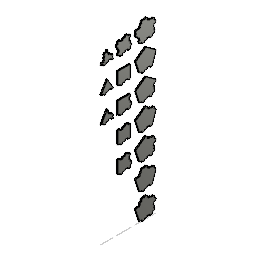
Test Game Pieces v1 (Autodesk Fusion 360 design; units mm, degrees)
Autodesk Fusion 360 part; units mm, degrees
sketch "Sketch1" plane through (0, 0, 0) normal (1, 0, 0) x (0, 0, -1)
  line L0 (0, 0) -> (10, 0)
  line L1 (5, 0) -> (5, 1)
  line L2 (5, 1) -> (5, 15)
  line L3 (10, 0) -> (5, 8.6603)
  line L4 (5, 8.6603) -> (0, 0)
  dimension "d1" = 10
  dimension "d2" = 10
  constraint coincident L0.start L4.end
  constraint horizontal L0
  constraint midpoint L0 L1.start
  constraint perpendicular L0 L1
  constraint perpendicular L0 L2
  constraint coincident L2 L3.end
  measures "d1" distance of L0.start L0.end
  measures "d2" distance of L0.end L3.end
extrude "Extrude1" add sketch "Sketch1" along normal blind 1 makes body 1
sketch "Sketch2" plane through (0, 0, 0) normal (1, 0, 0) x (0, 0, -1)
  line L0 (15, 0) -> (25, 0)
  line L1 (25, 0) -> (25, 10)
  line L2 (25, 10) -> (15, 10)
  line L3 (15, 10) -> (15, 0)
  dimension "d5" = 10
  dimension "d6" = 10
  constraint horizontal L0
  constraint vertical L1
  constraint horizontal L2
  constraint vertical L3
  measures "d5" distance of L0.start L0.end
  measures "d6" distance of L0.start L2.end
extrude "Extrude2" add sketch "Sketch2" along normal blind 1 separate body makes body 2
sketch "Sketch3" plane through (0, 0, 0) normal (1, 0, 0) x (0, 0, -1)
  line L0 (30, 0) -> (40, 0)
  line L1 (40, 0) -> (43.0902, 9.5106)
  line L2 (40, 0) -> (50, 0) construction
  line L3 (43.0902, 9.5106) -> (35, 15.3884)
  line L4 (43.0902, 9.5106) -> (53.0902, 9.5106) construction
  line L5 (30, 0) -> (26.9098, 9.5106)
  line L6 (30, 0) -> (40, 0) construction
  line L7 (26.9098, 9.5106) -> (35, 15.3884)
  dimension "d9" = 10
  dimension "d10" = 72
  dimension "d11" = 10
  dimension "d12" = 144
  dimension "d13" = 10
  dimension "d14" = 108
  dimension "d15" = 10
  constraint horizontal L0
  constraint horizontal L2
  constraint horizontal L4
  constraint horizontal L6
  measures "d9" distance of L0.start L0.end
  measures "d10" angle of L1 L2
  measures "d11" distance of L0.end L1.end
  measures "d12" angle of L3 L4
  measures "d13" distance of L1.end L3.end
  measures "d14" angle of L5 L6
  measures "d15" distance of L0.start L5.end
extrude "Extrude3" add sketch "Sketch3" along normal blind 1 separate body makes body 3
move_body "Move1" bodies 2 to x (1, 0, 0) y (0, 1, 0) z (0, 0, 1) at (0, 0, 2)
sketch "Sketch4" plane through (1, 0, 0) normal (1, 0, 0) x (0, 0, -1)
  line L0 (5, 8.6603) -> (0, 0)
  line L1 (0, 0) -> (10, 0)
  line L2 (10, 0) -> (5, 8.6603)
  line L3 (5, 0) -> (6, 0)
  line L4 (5, 0) -> (4, 0)
  line L5 (4, 0) -> (2, 0)
  line L6 (2, 0) -> (2, -1)
  line L7 (2, -1) -> (4, -1)
  line L8 (4, -1) -> (4, 0)
  line L9 (6, 0) -> (8, 0)
  line L10 (8, 0) -> (8, 1)
  line L11 (8, 1) -> (6, 1)
  line L12 (6, 1) -> (6, 0)
  line L13 (7.5, 4.3301) -> (8, 3.4641)
  line L14 (7.5, 4.3301) -> (7, 5.1962)
  line L15 (7, 5.1962) -> (6.134, 4.6962)
  line L16 (7, 5.1962) -> (6, 6.9282)
  line L17 (6, 6.9282) -> (5.134, 6.4282)
  line L18 (5.134, 6.4282) -> (6.134, 4.6962)
  line L19 (8, 3.4641) -> (8.866, 3.9641)
  line L20 (8.866, 3.9641) -> (9.866, 2.2321)
  line L21 (9.866, 2.2321) -> (9, 1.7321)
  line L22 (2.5, 4.3301) -> (3, 5.1962)
  line L23 (3, 5.1962) -> (2.134, 5.6962)
  line L24 (2.134, 5.6962) -> (3.134, 7.4282)
  line L25 (3.134, 7.4282) -> (4, 6.9282)
  line L26 (2.5, 4.3301) -> (2, 3.4641)
  line L27 (2, 3.4641) -> (2.866, 2.9641)
  line L28 (2.866, 2.9641) -> (1.866, 1.2321)
  line L29 (1.866, 1.2321) -> (1, 1.7321)
  dimension "d18" = 1
  dimension "d19" = 1
  dimension "d20" = 1
  dimension "d21" = 2
  dimension "d22" = 1
  dimension "d23" = 1
  dimension "d24" = 1
  dimension "d25" = 1
  dimension "d26" = 2
  dimension "d27" = 1
  dimension "d28" = 1
  dimension "d29" = 2
  dimension "d30" = 1
  dimension "d31" = 1
  dimension "d32" = 2
  dimension "d33" = 1
  dimension "d34" = 1
  dimension "d35" = 2
  constraint midpoint L1 L3.start
  constraint parallel L1 L3
  constraint parallel L1 L4
  constraint horizontal L5
  constraint vertical L6
  constraint horizontal L7
  constraint vertical L8
  constraint horizontal L9
  constraint vertical L10
  constraint horizontal L11
  constraint vertical L12
  constraint midpoint L2 L13.start
  constraint parallel L2 L13
  constraint parallel L2 L14
  constraint perpendicular L2 L15
  constraint perpendicular L15 L16
  constraint perpendicular L2 L17
  constraint perpendicular L13 L19
  constraint perpendicular L19 L20
  constraint coincident L2 L21.end
  constraint perpendicular L2 L21
  constraint midpoint L0 L22.start
  constraint parallel L0 L22
  constraint perpendicular L0 L23
  constraint perpendicular L23 L24
  constraint coincident L0 L25.end
  constraint perpendicular L0 L25
  constraint perpendicular L23 L26
  constraint perpendicular L0 L27
  constraint perpendicular L27 L28
  constraint coincident L0 L29.end
  constraint perpendicular L0 L29
  measures "d18" distance of L3.start L3.end
  measures "d19" distance of L3.start L4.end
  measures "d20" distance of L4.end L7.end
  measures "d21" distance of L3.end L9.end
  measures "d22" distance of L3.end L11.end
  measures "d23" distance of L13.start L13.end
  measures "d24" distance of L13.start L14.end
  measures "d25" distance of L14.end L15.end
  measures "d26" distance of L14.end L16.end
  measures "d27" distance of L16.end L17.end
  measures "d28" distance of L13.end L19.end
  measures "d29" distance of L19.end L20.end
  measures "d30" distance of L22.start L22.end
  measures "d31" distance of L22.end L23.end
  measures "d32" distance of L23.end L24.end
  measures "d33" distance of L22.start L26.end
  measures "d34" distance of L26.end L27.end
  measures "d35" distance of L27.end L28.end
extrude "Extrude4" add sketch "Sketch4" against normal blind 1 contours L1 L5 L6 L7 L8 bodies 1
extrude "Extrude5" cut sketch "Sketch4" against normal blind 1 contours L1 L9 L10 L11 L12 bodies 1
copy_body "CopyPasteBodies1" bodies 1 makes body 4
move_body "Move2" bodies 4 to x (1, 0, 0) y (0, 1, 0) z (0, 0, 1) at (0, -20, 0)
extrude "Extrude6" cut sketch "Sketch4" against normal blind 1 contours L2 L15 L16 L17 L18 bodies 1
extrude "Extrude7" add sketch "Sketch4" against normal blind 1 contours L2 L19 L20 L21 bodies 1
copy_body "CopyPasteBodies2" bodies 1 makes body 5
move_body "Move3" bodies 5 to x (1, 0, 0) y (0, 1, 0) z (0, 0, 1) at (0, -40, 0)
extrude "Extrude8" cut sketch "Sketch4" against normal blind 1 contours L0 L27 L28 L29 bodies 1
extrude "Extrude9" add sketch "Sketch4" against normal blind 1 contours L0 L23 L24 L25 bodies 1
sketch "Sketch5" plane through (1, 0, 0) normal (1, 0, 0) x (0, 0, -1)
  line L0 (13, 10) -> (13, 0)
  line L1 (13, 0) -> (23, 0)
  line L2 (23, 0) -> (23, 10)
  line L3 (23, 10) -> (13, 10)
  line L4 (18, 0) -> (19, 0)
  line L5 (19, 0) -> (21, 0)
  line L6 (21, 0) -> (21, 1)
  line L7 (21, 1) -> (19, 1)
  line L8 (19, 1) -> (19, 0)
  line L9 (18, 0) -> (17, 0)
  line L10 (17, 0) -> (15, 0)
  line L11 (15, 0) -> (15, -1)
  line L12 (15, -1) -> (17, -1)
  line L13 (17, -1) -> (17, 0)
  line L14 (23, 5) -> (23, 4)
  line L15 (23, 4) -> (24, 4)
  line L16 (24, 4) -> (24, 2)
  line L17 (24, 2) -> (23, 2)
  line L18 (23, 2) -> (23, 4)
  line L19 (23, 5) -> (23, 6)
  line L20 (23, 6) -> (22, 6)
  line L21 (22, 6) -> (22, 8)
  line L22 (22, 8) -> (23, 8)
  line L23 (23, 8) -> (23, 6)
  line L24 (18, 10) -> (19, 10)
  line L25 (19, 10) -> (21, 10)
  line L26 (21, 10) -> (21, 11)
  line L27 (21, 11) -> (19, 11)
  line L28 (19, 11) -> (19, 10)
  line L29 (18, 10) -> (17, 10)
  line L30 (17, 10) -> (15, 10)
  line L31 (15, 10) -> (15, 9)
  line L32 (15, 9) -> (17, 9)
  line L33 (17, 9) -> (17, 10)
  line L34 (13, 5) -> (13, 6)
  line L35 (13, 6) -> (12, 6)
  line L36 (12, 6) -> (12, 8)
  line L37 (12, 8) -> (13, 8)
  line L38 (13, 8) -> (13, 6)
  line L39 (13, 5) -> (13, 4)
  line L40 (13, 4) -> (14, 4)
  line L41 (14, 4) -> (14, 2)
  line L42 (14, 2) -> (13, 2)
  line L43 (13, 2) -> (13, 4)
  dimension "d48" = 1
  dimension "d49" = 2
  dimension "d50" = 1
  dimension "d51" = 1
  dimension "d52" = 2
  dimension "d53" = 1
  dimension "d54" = 1
  dimension "d55" = 1
  dimension "d56" = 2
  dimension "d57" = 1
  dimension "d58" = 1
  dimension "d59" = 2
  dimension "d60" = 1
  dimension "d61" = 2
  dimension "d62" = 1
  dimension "d63" = 1
  dimension "d64" = 2
  dimension "d65" = 1
  dimension "d66" = 1
  dimension "d67" = 1
  dimension "d68" = 2
  dimension "d69" = 1
  dimension "d70" = 1
  dimension "d71" = 2
  constraint midpoint L1 L4.start
  constraint parallel L1 L4
  constraint horizontal L5
  constraint vertical L6
  constraint horizontal L7
  constraint vertical L8
  constraint parallel L1 L9
  constraint horizontal L10
  constraint vertical L11
  constraint horizontal L12
  constraint vertical L13
  constraint midpoint L2 L14.start
  constraint parallel L2 L14
  constraint horizontal L15
  constraint vertical L16
  constraint horizontal L17
  constraint vertical L18
  constraint parallel L2 L19
  constraint horizontal L20
  constraint vertical L21
  constraint horizontal L22
  constraint vertical L23
  constraint midpoint L3 L24.start
  constraint parallel L3 L24
  constraint horizontal L25
  constraint vertical L26
  constraint horizontal L27
  constraint vertical L28
  constraint parallel L3 L29
  constraint horizontal L30
  constraint vertical L31
  constraint horizontal L32
  constraint vertical L33
  constraint midpoint L0 L34.start
  constraint parallel L0 L34
  constraint horizontal L35
  constraint vertical L36
  constraint horizontal L37
  constraint vertical L38
  constraint parallel L0 L39
  constraint horizontal L40
  constraint vertical L41
  constraint horizontal L42
  constraint vertical L43
  measures "d48" distance of L4.start L4.end
  measures "d49" distance of L4.end L5.end
  measures "d50" distance of L4.end L7.end
  measures "d51" distance of L4.start L9.end
  measures "d52" distance of L9.end L10.end
  measures "d53" distance of L9.end L12.end
  measures "d54" distance of L14.start L14.end
  measures "d55" distance of L14.end L15.end
  measures "d56" distance of L14.end L17.end
  measures "d57" distance of L14.start L19.end
  measures "d58" distance of L19.end L20.end
  measures "d59" distance of L19.end L22.end
  measures "d60" distance of L24.start L24.end
  measures "d61" distance of L24.end L25.end
  measures "d62" distance of L24.end L27.end
  measures "d63" distance of L24.start L29.end
  measures "d64" distance of L29.end L30.end
  measures "d65" distance of L29.end L32.end
  measures "d66" distance of L34.start L34.end
  measures "d67" distance of L34.end L35.end
  measures "d68" distance of L34.end L37.end
  measures "d69" distance of L34.start L39.end
  measures "d70" distance of L39.end L40.end
  measures "d71" distance of L39.end L42.end
extrude "Extrude10" add sketch "Sketch5" against normal blind 1 contours L1 L10 L11 L12 L13 bodies 2
extrude "Extrude11" cut sketch "Sketch5" against normal blind 1 contours L1 L5 L6 L7 L8 bodies 2
copy_body "CopyPasteBodies3" bodies 2 makes body 6
move_body "Move4" bodies 6 to x (1, 0, 0) y (0, 1, 0) z (0, 0, 1) at (0, -20, 0)
extrude "Extrude12" cut sketch "Sketch5" against normal blind 1 contours L2 L20 L21 L22 L23 bodies 2
extrude "Extrude13" add sketch "Sketch5" against normal blind 1 contours L2 L15 L16 L17 L18 bodies 2
copy_body "CopyPasteBodies4" bodies 2 makes body 7
move_body "Move5" bodies 7 to x (1, 0, 0) y (0, 1, 0) z (0, 0, 1) at (0, -40, 0)
extrude "Extrude14" cut sketch "Sketch5" against normal blind 1 contours L2 L15 L16 L17 L18 bodies 2
extrude "Extrude15" add sketch "Sketch5" against normal blind 1 contours L2 L20 L21 L22 L23 bodies 2
extrude "Extrude16" add sketch "Sketch5" against normal blind 1 contours L3 L25 L26 L27 L28 bodies 2
extrude "Extrude17" cut sketch "Sketch5" against normal blind 1 contours L3 L30 L31 L32 L33 bodies 2
copy_body "CopyPasteBodies5" bodies 2 makes body 8
move_body "Move6" bodies 8 to x (1, 0, 0) y (0, 1, 0) z (0, 0, 1) at (0, -60, 0)
extrude "Extrude18" add sketch "Sketch5" against normal blind 1 contours L3 L30 L31 L32 L33 bodies 2
extrude "Extrude19" cut sketch "Sketch5" against normal blind 1 contours L3 L25 L26 L27 L28 bodies 2
extrude "Extrude20" add sketch "Sketch5" against normal blind 1 contours L0 L35 L36 L37 L38 bodies 2
extrude "Extrude21" cut sketch "Sketch5" against normal blind 1 contours L0 L40 L41 L42 L43 bodies 2
extrude "Extrude22" cut sketch "Sketch5" against normal blind 1 contours L0 L35 L36 L37 L38 | L2 L20 L21 L22 L23 bodies 2
extrude "Extrude23" add sketch "Sketch5" against normal blind 1 contours L0 L40 L41 L42 L43 | L2 L15 L16 L17 L18 bodies 2
extrude "Extrude24" cut sketch "Sketch5" against normal blind 1 contours L3 L30 L31 L32 L33 bodies 2
extrude "Extrude25" add sketch "Sketch5" against normal blind 1 contours L3 L25 L26 L27 L28 bodies 2
copy_body "CopyPasteBodies7" bodies 2 makes body 9
move_body "Move8" bodies 9 to x (1, 0, 0) y (0, 1, 0) z (0, 0, 1) at (0, -100, 0)
extrude "Extrude26" cut sketch "Sketch5" against normal blind 1 contours L0 L40 L41 L42 L43 | L2 L15 L16 L17 L18 bodies 2
extrude "Extrude27" add sketch "Sketch5" against normal blind 1 contours L0 L35 L36 L37 L38 | L2 L20 L21 L22 L23 bodies 2
extrude "Extrude28" cut sketch "Sketch5" against normal blind 1 contours L2 L20 L21 L22 L23 | L2 L15 L16 L17 L18 bodies 2
extrude "Extrude29" add sketch "Sketch5" against normal blind 1 contours L2 L15 L16 L17 L18 bodies 2
move_body "Move11" bodies 9 to x (1, 0, 0) y (0, 1, 0) z (0, 0, 1) at (0, 20, 0)
sketch "Sketch6" plane through (1, 0, 0) normal (1, 0, 0) x (0, 0, -1)
  line L0 (30, 0) -> (40, 0)
  line L1 (40, 0) -> (43.0902, 9.5106)
  line L2 (43.0902, 9.5106) -> (35, 15.3884)
  line L3 (35, 15.3884) -> (26.9098, 9.5106)
  line L4 (26.9098, 9.5106) -> (30, 0)
  line L5 (35, 0) -> (36, 0)
  line L6 (36, 0) -> (36, 1)
  line L7 (36, 1) -> (38, 1)
  line L8 (38, 1) -> (38, 0)
  line L9 (35, 0) -> (34, 0)
  line L10 (34, 0) -> (34, -1)
  line L11 (34, -1) -> (32, -1)
  line L12 (32, -1) -> (32, 0)
  line L13 (41.5451, 4.7553) -> (41.8541, 5.7063)
  line L14 (41.8541, 5.7063) -> (40.903, 6.0154)
  line L15 (40.903, 6.0154) -> (41.5211, 7.9175)
  line L16 (41.5211, 7.9175) -> (42.4721, 7.6085)
  line L17 (41.5451, 4.7553) -> (41.2361, 3.8042)
  line L18 (41.2361, 3.8042) -> (42.1871, 3.4952)
  line L19 (42.1871, 3.4952) -> (41.5691, 1.5931)
  line L20 (41.5691, 1.5931) -> (40.618, 1.9021)
  line L21 (39.0451, 12.4495) -> (39.8541, 11.8617)
  line L22 (39.8541, 11.8617) -> (40.4419, 12.6707)
  line L23 (40.4419, 12.6707) -> (42.0599, 11.4952)
  line L24 (42.0599, 11.4952) -> (41.4721, 10.6861)
  line L25 (39.0451, 12.4495) -> (38.2361, 13.0373)
  line L26 (38.2361, 13.0373) -> (37.6483, 12.2283)
  line L27 (37.6483, 12.2283) -> (36.0302, 13.4038)
  line L28 (36.0302, 13.4038) -> (36.618, 14.2128)
  line L29 (30.9549, 12.4495) -> (31.7639, 13.0373)
  line L30 (31.7639, 13.0373) -> (31.1761, 13.8463)
  line L31 (31.1761, 13.8463) -> (32.7942, 15.0219)
  line L32 (32.7942, 15.0219) -> (33.382, 14.2128)
  line L33 (30.9549, 12.4495) -> (30.1459, 11.8617)
  line L34 (30.1459, 11.8617) -> (30.7337, 11.0527)
  line L35 (30.7337, 11.0527) -> (29.1156, 9.8771)
  line L36 (29.1156, 9.8771) -> (28.5279, 10.6861)
  line L37 (28.4549, 4.7553) -> (28.1459, 5.7063)
  line L38 (28.1459, 5.7063) -> (27.1948, 5.3973)
  line L39 (27.1948, 5.3973) -> (26.5768, 7.2994)
  line L40 (26.5768, 7.2994) -> (27.5279, 7.6085)
  line L41 (28.4549, 4.7553) -> (28.7639, 3.8042)
  line L42 (28.7639, 3.8042) -> (29.715, 4.1132)
  line L43 (29.715, 4.1132) -> (30.333, 2.2111)
  line L44 (30.333, 2.2111) -> (29.382, 1.9021)
  dimension "d112" = 2
  dimension "d113" = 2
  dimension "d114" = 1
  dimension "d115" = 1
  dimension "d116" = 2
  dimension "d117" = 1
  dimension "d118" = 1
  dimension "d119" = 2
  dimension "d120" = 1
  dimension "d121" = 1
  dimension "d122" = 2
  dimension "d123" = 1
  dimension "d124" = 1
  dimension "d125" = 2
  dimension "d126" = 1
  dimension "d127" = 1
  dimension "d128" = 2
  dimension "d129" = 1
  dimension "d130" = 1
  dimension "d131" = 2
  dimension "d132" = 1
  dimension "d133" = 1
  dimension "d134" = 2
  dimension "d135" = 1
  dimension "d136" = 1
  dimension "d137" = 2
  constraint midpoint L0 L5.start
  constraint coincident L0 L5.end
  constraint parallel L0 L5
  constraint perpendicular L5 L6
  constraint perpendicular L6 L7
  constraint coincident L0 L8.end
  constraint perpendicular L0 L8
  constraint coincident L0 L9.end
  constraint perpendicular L6 L9
  constraint perpendicular L0 L10
  constraint perpendicular L10 L11
  constraint coincident L0 L12.end
  constraint perpendicular L0 L12
  constraint midpoint L1 L13.start
  constraint parallel L1 L13
  constraint perpendicular L1 L14
  constraint perpendicular L14 L15
  constraint coincident L1 L16.end
  constraint perpendicular L1 L16
  constraint perpendicular L16 L17
  constraint perpendicular L17 L18
  constraint perpendicular L18 L19
  constraint coincident L1 L20.end
  constraint perpendicular L1 L20
  constraint midpoint L2 L21.start
  constraint parallel L2 L21
  constraint perpendicular L21 L22
  constraint perpendicular L22 L23
  constraint coincident L2 L24.end
  constraint perpendicular L2 L24
  constraint perpendicular L24 L25
  constraint perpendicular L2 L26
  constraint perpendicular L26 L27
  constraint coincident L2 L28.end
  constraint perpendicular L2 L28
  constraint midpoint L3 L29.start
  constraint parallel L3 L29
  constraint perpendicular L29 L30
  constraint perpendicular L30 L31
  constraint coincident L3 L32.end
  constraint perpendicular L3 L32
  constraint perpendicular L32 L33
  constraint perpendicular L33 L34
  constraint perpendicular L34 L35
  constraint coincident L3 L36.end
  constraint perpendicular L3 L36
  constraint midpoint L4 L37.start
  constraint parallel L4 L37
  constraint perpendicular L37 L38
  constraint perpendicular L38 L39
  constraint coincident L4 L40.end
  constraint perpendicular L4 L40
  constraint perpendicular L40 L41
  constraint perpendicular L4 L42
  constraint perpendicular L42 L43
  constraint coincident L4 L44.end
  constraint perpendicular L4 L44
  measures "d112" distance of L6.end L7.end
  measures "d113" distance of L10.end L11.end
  measures "d114" distance of L13.start L13.end
  measures "d115" distance of L13.end L14.end
  measures "d116" distance of L14.end L15.end
  measures "d117" distance of L13.start L17.end
  measures "d118" distance of L17.end L18.end
  measures "d119" distance of L18.end L19.end
  measures "d120" distance of L21.start L21.end
  measures "d121" distance of L21.end L22.end
  measures "d122" distance of L22.end L23.end
  measures "d123" distance of L21.start L25.end
  measures "d124" distance of L25.end L26.end
  measures "d125" distance of L26.end L27.end
  measures "d126" distance of L29.start L29.end
  measures "d127" distance of L29.end L30.end
  measures "d128" distance of L30.end L31.end
  measures "d129" distance of L29.start L33.end
  measures "d130" distance of L33.end L34.end
  measures "d131" distance of L34.end L35.end
  measures "d132" distance of L37.start L37.end
  measures "d133" distance of L37.end L38.end
  measures "d134" distance of L38.end L39.end
  measures "d135" distance of L37.start L41.end
  measures "d136" distance of L41.end L42.end
  measures "d137" distance of L42.end L43.end
extrude "Extrude30" add sketch "Sketch6" against normal blind 1 contours L0 L10 L11 L12 bodies 3
extrude "Extrude31" cut sketch "Sketch6" against normal blind 1 contours L0 L6 L7 L8 bodies 3
copy_body "CopyPasteBodies10" bodies 3 makes body 10
move_body "Move13" bodies 10 to x (1, 0, 0) y (0, 1, 0) z (0, 0, 1) at (0, -20, 0)
extrude "Extrude32" cut sketch "Sketch6" against normal blind 1 contours L1 L18 L19 L20 | L1 L14 L15 L16 bodies 3
extrude "Extrude33" add sketch "Sketch6" against normal blind 1 contours L1 L18 L19 L20 bodies 3
copy_body "CopyPasteBodies11" bodies 3 makes body 11
move_body "Move14" bodies 11 to x (1, 0, 0) y (0, 1, 0) z (0, 0, 1) at (0, -40, 0)
extrude "Extrude34" cut sketch "Sketch6" against normal blind 1 contours L1 L18 L19 L20 | L1 L14 L15 L16 | L2 L26 L27 L28 bodies 3
extrude "Extrude35" add sketch "Sketch6" against normal blind 1 contours L1 L14 L15 L16 | L2 L22 L23 L24 bodies 3
copy_body "CopyPasteBodies12" bodies 3 makes body 12
move_body "Move15" bodies 12 to x (1, 0, 0) y (0, 1, 0) z (0, 0, 1) at (0, -60, 0)
extrude "Extrude36" add sketch "Sketch6" against normal blind 1 contours L1 L18 L19 L20 bodies 3
extrude "Extrude37" cut sketch "Sketch6" against normal blind 1 contours L1 L14 L15 L16 bodies 3
copy_body "CopyPasteBodies13" bodies 3 makes body 13
move_body "Move16" bodies 13 to x (1, 0, 0) y (0, 1, 0) z (0, 0, 1) at (0, -80, 0)
extrude "Extrude38" cut sketch "Sketch6" against normal blind 1 contours L1 L18 L19 L20 | L3 L34 L35 L36 bodies 3
extrude "Extrude39" add sketch "Sketch6" against normal blind 1 contours L1 L14 L15 L16 | L3 L30 L31 L32 bodies 3
copy_body "CopyPasteBodies14" bodies 3 makes body 14
move_body "Move17" bodies 14 to x (1, 0, 0) y (0, 1, 0) z (0, 0, 1) at (0, -100, 0)
extrude "Extrude40" cut sketch "Sketch6" against normal blind 1 contours L1 L14 L15 L16 bodies 3
extrude "Extrude41" add sketch "Sketch6" against normal blind 1 contours L1 L18 L19 L20 bodies 3
copy_body "CopyPasteBodies15" bodies 3 makes body 15
move_body "Move18" bodies 15 to x (1, 0, 0) y (0, 1, 0) z (0, 0, 1) at (0, -120, 0)
extrude "Extrude42" cut sketch "Sketch6" against normal blind 1 contours L4 L42 L43 L44 bodies 3
extrude "Extrude43" add sketch "Sketch6" against normal blind 1 contours L4 L38 L39 L40 bodies 3
equation "d10 = 180.0 deg - 108 deg"
named bodies: "Tri-3", "Squ-4", "Pen-5", "Tri-1", "Tri-2", "Squ-1", "Squ-2a", "Squ-2b", "Squ-3", "Pen-1", "Pen-2a", "Pen-2b", "Pen-3a", "Pen-3b", "Pen-4"
